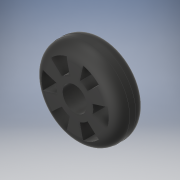
# Autodesk Inventor part: Wheel
Saved by Autodesk Inventor 2017 SP1 (Build 210196100, 196)
## iProperties
Created: 2018-02-11
Part Number: Wheel
Material: ABS Plastic
Document SubType Name: Modeling
Designer: Zach
Density: 1.06 g/cm^3
Appearance: Smooth - Black
Author: Zach
Autodesk Inventor part; units mm, degrees
ref_plane "YZ Plane" through (0, 0, 0) normal (1, 0, 0) x (0, 1, 0)
ref_plane "XZ Plane" through (0, 0, 0) normal (0, 1, 0) x (-1, 0, 0)
ref_plane "XY Plane" through (0, 0, 0) normal (0, 0, 1) x (1, 0, 0)
sketch "Sketch1" plane through (0, 0, 0) normal (0, 0, 1) x (1, 0, 0)
  circle A0 centre (0, 0) radius 2
  circle A1 centre (0, 0) radius 7
  circle A2 centre (0, 0) radius 3 construction
  circle A3 centre (0, 0) radius 5.5 construction
  line L0 (2.9047, 0.75) -> (5.2915, 1.5)
  line L1 (2.9047, -0.75) -> (5.2915, -1.5)
  arc A4 (2.9047, -0.75) -> (2.9047, 0.75) centre (0, 0) ccw
  arc A5 (5.2915, -1.5) -> (5.2915, 1.5) centre (0, 0) ccw
  line L2 (0, 0) -> (8.9421, 0) construction
  circle A6 centre (0, 0) radius 3 construction
  circle A7 centre (0, 0) radius 5.5 construction
  line L3 (0.8028, 2.8906) -> (1.3467, 5.3326)
  line L4 (2.1019, 2.1406) -> (3.9448, 3.8326)
  arc A8 (2.1019, 2.1406) -> (0.8028, 2.8906) centre (0, 0) ccw
  arc A9 (3.9448, 3.8326) -> (1.3467, 5.3326) centre (0, 0) ccw
  line L5 (0, 0) -> (4.471, 7.7441) construction
  circle A10 centre (0, 0) radius 3 construction
  circle A11 centre (0, 0) radius 5.5 construction
  line L6 (-2.1019, 2.1406) -> (-3.9448, 3.8326)
  line L7 (-0.8028, 2.8906) -> (-1.3467, 5.3326)
  arc A12 (-0.8028, 2.8906) -> (-2.1019, 2.1406) centre (0, 0) ccw
  arc A13 (-1.3467, 5.3326) -> (-3.9448, 3.8326) centre (0, 0) ccw
  line L8 (0, 0) -> (-4.471, 7.7441) construction
  circle A14 centre (0, 0) radius 3 construction
  circle A15 centre (0, 0) radius 5.5 construction
  line L9 (-2.9047, -0.75) -> (-5.2915, -1.5)
  line L10 (-2.9047, 0.75) -> (-5.2915, 1.5)
  arc A16 (-2.9047, 0.75) -> (-2.9047, -0.75) centre (0, 0) ccw
  arc A17 (-5.2915, 1.5) -> (-5.2915, -1.5) centre (0, 0) ccw
  line L11 (0, 0) -> (-8.9421, 0) construction
  circle A18 centre (0, 0) radius 3 construction
  circle A19 centre (0, 0) radius 5.5 construction
  line L12 (-0.8028, -2.8906) -> (-1.3467, -5.3326)
  line L13 (-2.1019, -2.1406) -> (-3.9448, -3.8326)
  arc A20 (-2.1019, -2.1406) -> (-0.8028, -2.8906) centre (0, 0) ccw
  arc A21 (-3.9448, -3.8326) -> (-1.3467, -5.3326) centre (0, 0) ccw
  line L14 (0, 0) -> (-4.471, -7.7441) construction
  circle A22 centre (0, 0) radius 3 construction
  circle A23 centre (0, 0) radius 5.5 construction
  line L15 (2.1019, -2.1406) -> (3.9448, -3.8326)
  line L16 (0.8028, -2.8906) -> (1.3467, -5.3326)
  arc A24 (0.8028, -2.8906) -> (2.1019, -2.1406) centre (0, 0) ccw
  arc A25 (1.3467, -5.3326) -> (3.9448, -3.8326) centre (0, 0) ccw
  line L17 (0, 0) -> (4.471, -7.7441) construction
  dimension "d0" = 4
  dimension "d1" = 14
  dimension "d2" = 6
  dimension "d3" = 11
  dimension "d4" = 0.75
  dimension "d5" = 0.75
  dimension "d8" = 360
  constraints: 48 point on circle, 36 end point, 26 centre point, 9 coincident, 2 concentric, 1 horizontal, 98 other
  measures "d0" diameter of A0
  measures "d1" diameter of A1
  measures "d2" diameter of A2
  measures "d3" diameter of A3
  measures "d4" vertical distance of point (0, 0) L0.start
  measures "d5" vertical distance of L0.start L0.end
extrude "Extrusion1" add sketch "Sketch1" along normal blind 5
fillet "Fillet1" radius 2 2 edges at (-7, 0, 5) (-7, 0, 0)
body "Solid1"
